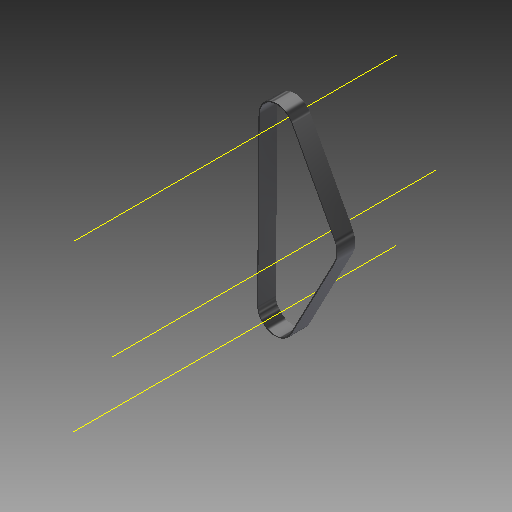
# Autodesk Inventor part: Synchronous Belt
Saved by Autodesk Inventor 2019.4 (Build 234330000, 330)
## iProperties
Created: 2020-01-06
Part Number: Synchronous Belt
Material: Rubber
Document SubType Name: Modeling
Designer: admin
Density: 1 g/cm^3
Appearance: Rubber - Black - Version 1.1
CustomPartVersion: 1
Author: admin
Autodesk Inventor part; units mm, degrees
sketch "Sketch Path" plane through (0, 0, 0) normal (0, 0, 1) x (1, 0, 0)
  arc A0 (-17.228958, -150.15559) -> (12.779623, -157.685828) centre (-1.314047, -150.291816) ccw
  arc A1 (14.008922, 7.495015) -> (-15.942575, 0.129426) centre (-0.027664, -0.0068) ccw
  arc A2 (52.225593, -82.498169) -> (52.154238, -63.878386) centre (34.608505, -73.255654) ccw
  line L0 (52.225593, -82.498169) -> (12.779623, -157.685828)
  line L1 (-17.228958, -150.15559) -> (-15.942575, 0.129426)
  line L2 (14.008922, 7.495015) -> (52.154238, -63.878386)
  constraints: 6 end point, 6 point on circle, 3 centre point
ref_plane "Cross Section Plane" through (12.779623, -157.685828, 0) normal (0.4645795, 0.8855314, 0) x (0, 0, 1)
ref_plane "Work Plane2" through (-1.314047, -150.291816, 0) normal (-1, 0, 0) x (0, 0, 1)
ref_plane "Work Plane3" through (-0.027664, -0.0068, 0) normal (-0.2916059, -0.9565385, 0) x (0, 0, 1)
ref_plane "Work Plane4" through (34.608505, -73.255654, 0) normal (-0.3992571, 0.916839, 0) x (0, 0, 1)
sketch "Cross Section" plane through (12.779623, -157.685828, 0) normal (0.4645795, 0.8855314, 0) x (0, 0, 1)
  line L0 (-8, 0.5) -> (8, 0.5)
  line L1 (8, 0.5) -> (8, -0.5)
  line L2 (8, -0.5) -> (-8, -0.5)
  line L3 (-8, -0.5) -> (-8, 0.5)
  line L4 (-8, 0) -> (8, 0) construction
  point P0 (0, 0)
  point P1 (0, 0)
  dimension "d0" = 16
  dimension "d4" = 0.5
  dimension "d5" = 0.5
  constraints: 10 end point, 3 midpoint, 2 parallel, 1 coincident, 1 horizontal, 1 perpendicular, 1 other
  measures "d0" distance between parallel lines of L1 L3
  measures "d4" distance between parallel lines of L2 L4
  measures "d5" distance between parallel lines of L4 L0
sweep "Belt" add profiles "Cross Section" path "Sketch Path" path curves L2 A2 L0 A0 L1 A1
equation "\"d0\" = da_B"
equation "\"d4\" = da_a"
equation "\"d5\" = da_a2"
equation "\"da_B\" = 16"
equation "\"da_pb\" = 5"
equation "\"da_a\" = 0.5"
equation "\"da_S\" = 2.65"
equation "\"da_Beta\" = 20deg"
equation "\"da_Ht\" = 1.2"
equation "\"da_H\" = 2.2"
equation "\"da_a2\" = 0.5"
body "Solid1"
